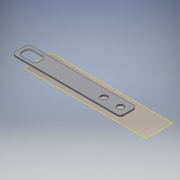
# Autodesk Inventor part: hangmount
Saved by Autodesk Inventor 2016 SP2 (Build 200236200, 236)
## iProperties
Created: 2018-10-04
Part Number: hangmount
Material: Generisch
Document SubType Name: Modeling
Designer: Nils
Density: 1 g/cm^3
Appearance: Vorgabe
Author: Nils
Autodesk Inventor part; units mm, degrees
ref_plane "YZ Plane" through (0, 0, 0) normal (1, 0, 0) x (0, 1, 0)
ref_plane "XZ Plane" through (0, 0, 0) normal (0, 1, 0) x (-1, 0, 0)
ref_plane "XY Plane" through (0, 0, 0) normal (0, 0, 1) x (1, 0, 0)
ref_plane "Arbeitsebene1" through (0, 0, 0) normal (0, 0, 1) x (1, 0, 0)
sketch "Skizze1" plane through (0, 0, 0) normal (0, 0, 1) x (1, 0, 0)
  circle A0 centre (118, -9.35) radius 5 construction
  circle A1 centre (118, -9.35) radius 5
  circle A2 centre (93, -9.35) radius 5 construction
  circle A3 centre (93, -9.35) radius 5
  line L0 (130.5, -21.85) -> (-35, -21.85)
  line L1 (-35, -21.85) -> (-35, 3.15)
  line L2 (-35, 3.15) -> (130.5, 3.15)
  line L3 (130.5, 3.15) -> (130.5, -21.85)
  line L4 (-30, -16.85) -> (-5, -16.85)
  line L5 (-5, -16.85) -> (-5, -1.85)
  line L6 (-5, -1.85) -> (-30, -1.85)
  line L7 (-30, -1.85) -> (-30, -16.85)
  line L8 (0, -2.2) -> (0, -28) construction
  point P0 (0, 0)
  dimension "d0" = 12.5
  dimension "d1" = 25
  dimension "d2" = 12.5
  dimension "d3" = 5
  dimension "d4" = 5
  dimension "d5" = 5
  dimension "d6" = 25
  dimension "d7" = 5
  dimension "d8" = 15
  constraints: 16 end point, 4 parallel, 2 centre point, 2 coincident, 2 concentric, 2 horizontal, 2 perpendicular
  measures "d0" distance from line of L0 A2.centre
  measures "d1" distance between parallel lines of L2 L0
  measures "d2" distance from line of A0.centre L3
  measures "d3" distance between parallel lines of L0 L4
  measures "d4" distance between parallel lines of L2 L6
  measures "d5" distance between parallel lines of L1 L7
  measures "d6" distance between parallel lines of L7 L5
  measures "d7" distance between parallel lines of L8 L5
  measures "d8" distance between parallel lines of L6 L4
extrude "Extrusion1" add sketch "Skizze1" along normal blind 2
fillet "Rundung1" radius 5 8 edges at (-5, -16.85, 1) (-30, -16.85, 1) (-30, -1.85, 1) (-5, -1.85, 1) (-35, -21.85, 1) (-35, 3.15, 1) (130.5, -21.85, 1) (130.5, 3.15, 1)
fillet "Rundung2" radius 1 16 edges at (-17.5, -1.85, 2) (-28.5355, -3.3145, 2) (-30, -9.35, 2) (-28.5355, -15.3855, 2) (-17.5, -16.85, 2) (-6.4645, -15.3855, 2) (-5, -9.35, 2) (-6.4645, -3.3145, 2) (-5, -9.35, 0) (-6.4645, -15.3855, 0) (-17.5, -16.85, 0) (-28.5355, -15.3855, 0) (-30, -9.35, 0) (-28.5355, -3.3145, 0) (-17.5, -1.85, 0) (-6.4645, -3.3145, 0)
equation "\"d1\" = 2 * d0"
equation "\"d2\" = d0"
equation "\"d4\" = d3"
equation "\"d5\" = d3"
equation "\"d7\" = d3"
